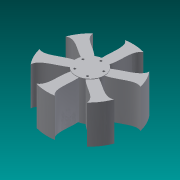
# Autodesk Inventor part: velg
Saved by Autodesk Inventor 2014 SP2 (Build 180246200, 246)
## iProperties
Created: 2019-07-22
Part Number: velg
Material: Aluminum 6061
Document SubType Name: Modeling
Designer: USER PC
Density: 2.71 g/cm^3
Appearance: Aluminum - Flat
Author: USER PC
Autodesk Inventor part; units mm, degrees
ref_plane "YZ Plane" through (0, 0, 0) normal (1, 0, 0) x (0, 1, 0)
ref_plane "XZ Plane" through (0, 0, 0) normal (0, 1, 0) x (-1, 0, 0)
sketch "Sketch2" plane through (0, 0, 0) normal (0, 0, 1) x (1, 0, 0)
  point P0 (0, 0)
ref_plane "Work Plane1" through (0, 0, 87.5) normal (0, 0, 1) x (1, 0, 0)
sketch "Sketch3" plane through (0, 0, 87.5) normal (0, 0, 1) x (1, 0, 0)
  circle A0 centre (0, 0) radius 65
  circle A1 centre (0, 50) radius 5
  circle A2 centre (-47.5528, 15.4508) radius 5
  circle A3 centre (-29.3893, -40.4508) radius 5
  circle A4 centre (29.3893, -40.4508) radius 5
  circle A5 centre (47.5528, 15.4508) radius 5
  dimension "d11" = 130
  dimension "d33" = 10
  dimension "d36" = 360
  constraints: 6 centre point, 1 coincident, 11 other
  measures "d11" diameter of A0
  measures "d33" diameter of A1
sketch "Sketch5" plane through (0, 0, 0) normal (0, 0, 1) x (1, 0, 0)
  circle A0 centre (0, 0) radius 30
  circle A1 centre (0, 0) radius 190.5
  line L0 (6.509, 17.129) -> (57.211, 63.0349) construction
  line L1 (57.211, 63.0349) -> (22.2678, 145.9394) construction
  line L2 (22.2678, 145.9394) -> (41.4523, 171.2904) construction
  line L3 (41.4523, 171.2904) -> (59.2665, 184.9937) construction
  spline S0 degree 4 poles (6.509, 17.129) (57.211, 63.0349) (22.2678, 145.9394) (41.4523, 171.2904) (59.2665, 184.9937) knots 1 1 1 1 1 2 2 2 2 2
  line L4 (0, 17.129) -> (-30, 60.9794) construction
  line L5 (-30, 60.9794) -> (0, 136.3472) construction
  line L6 (0, 136.3472) -> (-6.509, 176.0866) construction
  line L7 (-6.509, 176.0866) -> (-30, 190.5) construction
  spline S1 degree 4 poles (0, 17.129) (-30, 60.9794) (0, 136.3472) (-6.509, 176.0866) (-30, 190.5) knots 1 1 1 1 1 2 2 2 2 2
  line L8 (0, 17.129) -> (6.509, 17.129)
  arc A2 (59.2665, 184.9937) -> (-30, 190.5) centre (2.5103, -8.7844) ccw
  line L9 (-11.5797, 14.2015) -> (-25.9843, 81.0636) construction
  line L10 (-25.9843, 81.0636) -> (-115.2534, 92.2542) construction
  line L11 (-115.2534, 92.2542) -> (-127.6157, 121.5439) construction
  line L12 (-127.6157, 121.5439) -> (-130.576, 143.8231) construction
  spline S2 degree 4 poles (-11.5797, 14.2015) (-25.9843, 81.0636) (-115.2534, 92.2542) (-127.6157, 121.5439) (-130.576, 143.8231) knots 1 1 1 1 1 2 2 2 2 2
  line L13 (-14.8342, 8.5645) -> (-67.8097, 4.5089) construction
  line L14 (-67.8097, 4.5089) -> (-118.0801, 68.1736) construction
  line L15 (-118.0801, 68.1736) -> (-155.7499, 82.4063) construction
  line L16 (-155.7499, 82.4063) -> (-179.9778, 69.2692) construction
  spline S3 degree 4 poles (-14.8342, 8.5645) (-67.8097, 4.5089) (-118.0801, 68.1736) (-155.7499, 82.4063) (-179.9778, 69.2692) knots 1 1 1 1 1 2 2 2 2 2
  line L17 (-14.8342, 8.5645) -> (-11.5797, 14.2015)
  arc A3 (-130.576, 143.8231) -> (-179.9778, 69.2692) centre (8.8627, -2.2182) ccw
  line L18 (-18.0887, -2.9275) -> (-83.1953, 18.0287) construction
  line L19 (-83.1953, 18.0287) -> (-137.5211, -53.6853) construction
  line L20 (-137.5211, -53.6853) -> (-169.068, -49.7465) construction
  line L21 (-169.068, -49.7465) -> (-189.8425, -41.1705) construction
  spline S4 degree 4 poles (-18.0887, -2.9275) (-83.1953, 18.0287) (-137.5211, -53.6853) (-169.068, -49.7465) (-189.8425, -41.1705) knots 1 1 1 1 1 2 2 2 2 2
  line L22 (-14.8342, -8.5645) -> (-37.8097, -56.4705) construction
  line L23 (-37.8097, -56.4705) -> (-118.0801, -68.1736) construction
  line L24 (-118.0801, -68.1736) -> (-149.2409, -93.6803) construction
  line L25 (-149.2409, -93.6803) -> (-149.9778, -121.2308) construction
  spline S5 degree 4 poles (-14.8342, -8.5645) (-37.8097, -56.4705) (-118.0801, -68.1736) (-149.2409, -93.6803) (-149.9778, -121.2308) knots 1 1 1 1 1 2 2 2 2 2
  line L26 (-14.8342, -8.5645) -> (-18.0887, -2.9275)
  arc A4 (-189.8425, -41.1705) -> (-149.9778, -121.2308) centre (6.3524, 6.5662) ccw
  line L27 (-6.509, -17.129) -> (-57.211, -63.0349) construction
  line L28 (-57.211, -63.0349) -> (-22.2678, -145.9394) construction
  line L29 (-22.2678, -145.9394) -> (-41.4523, -171.2904) construction
  line L30 (-41.4523, -171.2904) -> (-59.2665, -184.9937) construction
  spline S6 degree 4 poles (-6.509, -17.129) (-57.211, -63.0349) (-22.2678, -145.9394) (-41.4523, -171.2904) (-59.2665, -184.9937) knots 1 1 1 1 1 2 2 2 2 2
  line L31 (0, -17.129) -> (30, -60.9794) construction
  line L32 (30, -60.9794) -> (0, -136.3472) construction
  line L33 (0, -136.3472) -> (6.509, -176.0866) construction
  line L34 (6.509, -176.0866) -> (30, -190.5) construction
  spline S7 degree 4 poles (0, -17.129) (30, -60.9794) (0, -136.3472) (6.509, -176.0866) (30, -190.5) knots 1 1 1 1 1 2 2 2 2 2
  line L35 (0, -17.129) -> (-6.509, -17.129)
  arc A5 (-59.2665, -184.9937) -> (30, -190.5) centre (-2.5103, 8.7844) ccw
  line L36 (11.5797, -14.2015) -> (25.9843, -81.0636) construction
  line L37 (25.9843, -81.0636) -> (115.2534, -92.2542) construction
  line L38 (115.2534, -92.2542) -> (127.6157, -121.5439) construction
  line L39 (127.6157, -121.5439) -> (130.576, -143.8231) construction
  spline S8 degree 4 poles (11.5797, -14.2015) (25.9843, -81.0636) (115.2534, -92.2542) (127.6157, -121.5439) (130.576, -143.8231) knots 1 1 1 1 1 2 2 2 2 2
  line L40 (14.8342, -8.5645) -> (67.8097, -4.5089) construction
  line L41 (67.8097, -4.5089) -> (118.0801, -68.1736) construction
  line L42 (118.0801, -68.1736) -> (155.7499, -82.4063) construction
  line L43 (155.7499, -82.4063) -> (179.9778, -69.2692) construction
  spline S9 degree 4 poles (14.8342, -8.5645) (67.8097, -4.5089) (118.0801, -68.1736) (155.7499, -82.4063) (179.9778, -69.2692) knots 1 1 1 1 1 2 2 2 2 2
  line L44 (14.8342, -8.5645) -> (11.5797, -14.2015)
  arc A6 (130.576, -143.8231) -> (179.9778, -69.2692) centre (-8.8627, 2.2182) ccw
  line L45 (18.0887, 2.9275) -> (83.1953, -18.0287) construction
  line L46 (83.1953, -18.0287) -> (137.5211, 53.6853) construction
  line L47 (137.5211, 53.6853) -> (169.068, 49.7465) construction
  line L48 (169.068, 49.7465) -> (189.8425, 41.1705) construction
  spline S10 degree 4 poles (18.0887, 2.9275) (83.1953, -18.0287) (137.5211, 53.6853) (169.068, 49.7465) (189.8425, 41.1705) knots 1 1 1 1 1 2 2 2 2 2
  line L49 (14.8342, 8.5645) -> (37.8097, 56.4705) construction
  line L50 (37.8097, 56.4705) -> (118.0801, 68.1736) construction
  line L51 (118.0801, 68.1736) -> (149.2409, 93.6803) construction
  line L52 (149.2409, 93.6803) -> (149.9778, 121.2308) construction
  spline S11 degree 4 poles (14.8342, 8.5645) (37.8097, 56.4705) (118.0801, 68.1736) (149.2409, 93.6803) (149.9778, 121.2308) knots 1 1 1 1 1 2 2 2 2 2
  line L53 (14.8342, 8.5645) -> (18.0887, 2.9275)
  arc A7 (189.8425, 41.1705) -> (149.9778, 121.2308) centre (-6.3524, -6.5662) ccw
  dimension "d24" = 60
  dimension "d25" = 381
  dimension "d28" = 360
  constraints: 12 end point, 12 point on circle, 8 centre point, 2 coincident, 175 other
  measures "d24" diameter of A0
  measures "d25" diameter of A1
extrude "Extrusion4" add sketch "Sketch5" along normal blind 175 contours S10 L53 S11 A0 | A0 S11 A1 S10 | S9 A1 S8 A0 | A0 S8 L44 S9 | A1 S11 A7 S10 | S9 A6 S8 A1 | S0 L8 S1 A0 | A0 S1 A1 S0 | S7 A1 S6 A0 | A0 S6 L35 S7 | A1 S1 A2 S0 | S7 A5 S6 A1 | S2 L17 S3 A0 | A0 S3 A1 S2 | S5 A1 S4 A0 | A0 S4 L26 S5 | A1 S3 A3 S2 | S5 A4 S4 A1
extrude "Extrusion5" add sketch "Sketch3" along normal mid plane 180
sketch "Sketch6" plane through (0, 0, -2.5) normal (0, 0, -1) x (-1, 0, 0)
  circle A0 centre (-47.5528, 15.4508) radius 5 projected
  circle A1 centre (-29.3893, -40.4508) radius 5 projected
  circle A2 centre (29.3893, -40.4508) radius 5 projected
  circle A3 centre (47.5528, 15.4508) radius 5 projected
  circle A4 centre (0, 50) radius 5 projected
  circle A5 centre (0, 0) radius 65 projected
  circle A6 centre (0, 50) radius 5
  circle A7 centre (-47.5528, 15.4508) radius 5
  circle A8 centre (-29.3893, -40.4508) radius 5
  circle A9 centre (29.3893, -40.4508) radius 5
  circle A10 centre (47.5528, 15.4508) radius 5
  dimension "d42" = 360
  constraints: 5 centre point, 1 coincident, 1 concentric, 11 other
extrude "Extrusion6" cut sketch "Sketch6" against normal blind 1800 contours A0 | A1 | A2 | A3 | A4
body "Solid1"
